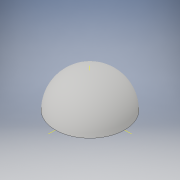
# Autodesk Inventor part: nosecone
Saved by Autodesk Inventor 2018 (Build 220112000, 112)
## iProperties
Created: 2018-04-21
Part Number: nosecone
Material: Generic
Document SubType Name: Modeling
Designer: atbin
Mass: 474963 g
Surface Area: 92839.4 cm^2
Volume: 2.04762e+06 cm^3
Density: 0.231958 g/cm^3
Appearance: Default
Author: atbin
Autodesk Inventor part; units mm, degrees
ref_plane "YZ Plane" through (0, 0, 0) normal (1, 0, 0) x (0, 1, 0)
ref_plane "XZ Plane" through (0, 0, 0) normal (0, 1, 0) x (-1, 0, 0)
ref_plane "XY Plane" through (0, 0, 0) normal (0, 0, 1) x (1, 0, 0)
sketch "Sketch2" plane through (0, 0, 0) normal (0, 1, 0) x (-1, 0, 0)
  arc A0 (-992.5, 0) -> (992.5, 0) centre (0, 0) ccw
  line L0 (992.5, 0) -> (-992.5, 0)
  dimension "d0" = 1985
  dimension "d0" = 1985
  constraints: 2 end point, 2 point on circle, 1 centre point, 1 coincident
  measures "d0" diameter of A0
revolve "Revolution1" add sketch "Sketch2" angle 180 about axis through (-992.5, 0, 0) along (1, 0, 0)
body "Solid1"
